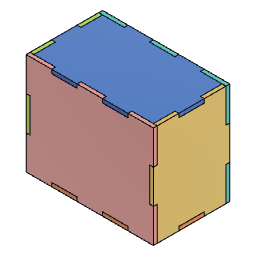
Box (Autodesk Fusion 360 design; units mm, degrees)
Autodesk Fusion 360 part; units mm, degrees
sketch "Sketch1" plane through (0, 0, 0) normal (0, 1, 0) x (1, 0, 0) in component "side 1"
  line L0 (0, 0) -> (100, 0)
  line L1 (100, 0) -> (100, -80)
  line L2 (100, -80) -> (0, -80)
  line L3 (0, -80) -> (0, 0)
  line L4 (3, 0) -> (3, -80) construction
  line L5 (0, -3) -> (100, -3) construction
  line L6 (20, 0) -> (40, 0)
  line L7 (40, 0) -> (40, -3)
  line L8 (40, -3) -> (20, -3)
  line L9 (20, -3) -> (20, 0)
  line L10 (60, 0) -> (80, 0)
  line L11 (80, 0) -> (80, -3)
  line L12 (80, -3) -> (60, -3)
  line L13 (60, -3) -> (60, 0)
  line L14 (0, -53.3333) -> (3, -53.3333)
  line L15 (3, -53.3333) -> (3, -26.6667)
  line L16 (3, -26.6667) -> (0, -26.6667)
  line L17 (0, -26.6667) -> (0, -53.3333)
  line L18 (50, -80) -> (50, -85.2851) construction
  line L19 (100, -40) -> (106.0423, -40) construction
  line L20 (100, -53.3333) -> (97, -53.3333)
  line L21 (97, -26.6667) -> (100, -26.6667)
  line L22 (97, -53.3333) -> (97, -26.6667)
  line L23 (97, 0) -> (97, -80) construction
  line L24 (100, -26.6667) -> (100, -53.3333)
  line L25 (80, -80) -> (80, -77)
  line L26 (20, -77) -> (20, -80)
  line L27 (20, -80) -> (40, -80)
  line L28 (0, -77) -> (100, -77) construction
  line L29 (40, -77) -> (20, -77)
  line L30 (60, -77) -> (60, -80)
  line L31 (60, -80) -> (80, -80)
  line L32 (40, -80) -> (40, -77)
  line L33 (80, -77) -> (60, -77)
  dimension "d7" = 80
  dimension "d8" = 100
  dimension "d9" = 3
  dimension "d10" = 3
  dimension "d11" = 20
  dimension "d12" = 20
  dimension "d13" = 20
  dimension "d14" = 20
  dimension "d15" = 26.6667
  dimension "d16" = 26.6667
  constraint horizontal L0
  constraint vertical L1
  constraint horizontal L2
  constraint vertical L3
  constraint coincident L0.start L3.end
  constraint coincident L0 L4.start
  constraint coincident L2 L4.end
  constraint perpendicular L2 L4
  constraint coincident L3 L5.start
  constraint coincident L1 L5.end
  constraint perpendicular L1 L5
  constraint horizontal L6
  constraint vertical L7
  constraint horizontal L8
  constraint vertical L9
  constraint coincident L5 L7.end
  constraint coincident L0 L6.start
  constraint horizontal L10
  constraint vertical L11
  constraint horizontal L12
  constraint vertical L13
  constraint coincident L5 L11.end
  constraint coincident L0 L10.start
  constraint horizontal L14
  constraint vertical L15
  constraint horizontal L16
  constraint vertical L17
  constraint coincident L4 L15.end
  constraint coincident L3 L14.start
  constraint midpoint L2 L18.start
  constraint perpendicular L2 L18
  constraint midpoint L1 L19.start
  constraint perpendicular L1 L19
  constraint symmetric L4.start L18 L23.start
  constraint symmetric L4.end L18 L23.end
  constraint symmetric L14.start L18 L20.start
  constraint symmetric L14.end L18 L20.end
  constraint symmetric L15.end L18 L21.start
  constraint symmetric L16.end L18 L21.end
  constraint symmetric L5.start L19 L28.start
  constraint symmetric L5.end L19 L28.end
  constraint symmetric L6.start L19 L26.end
  constraint symmetric L6.end L19 L27.end
  constraint symmetric L7.end L19 L29.start
  constraint symmetric L8.end L19 L26.start
  constraint symmetric L10.start L19 L30.end
  constraint symmetric L10.end L19 L25.start
  constraint symmetric L11.end L19 L25.end
  constraint symmetric L12.end L19 L30.start
  measures "d7" distance of L0.start L2.end
  measures "d8" distance of L0.start L0.end
  measures "d9" distance of L3 L4
  measures "d10" distance of L0 L5
  measures "d11" distance of L3 L9
  measures "d12" distance of L7 L9
  measures "d13" distance of L7 L13
  measures "d14" distance of L11 L13
  measures "d15" distance of L0 L16
  measures "d16" distance of L14 L16
extrude "Extrude1" add sketch "Sketch1" along normal blind 3 contours L0 L1 L2 L3 L7 L8 L9 L11 L12 L13 L14 L15 L16 L20 L21 L22 L25 L26 L29 L30 L32 L33 makes body 1 in component "side 1"
sketch "Sketch1 (2)" plane through (97, 0, 0) normal (1, 0, 0) x (0, 1, 0) in component "side 2"
  line L0 (0, 53.3333) -> (0, 26.6667)
  line L1 (0, 26.6667) -> (3, 26.6667)
  line L2 (3, 26.6667) -> (3, 53.3333)
  line L3 (3, 53.3333) -> (0, 53.3333)
  line L4 (0, 0) -> (60, 0)
  line L5 (60, 0) -> (60, 80)
  line L6 (60, 80) -> (0, 80)
  line L7 (0, 80) -> (0, 0)
  line L8 (0, 0) -> (3, 0)
  line L9 (0, 0) -> (0, 26.6667)
  line L10 (0, 80) -> (3, 80)
  line L11 (3, 80) -> (3, 0) construction
  line L12 (0, 3) -> (60, 3) construction
  line L13 (30, 80) -> (30, 85.6463) construction
  line L14 (60, 40) -> (65.0894, 40) construction
  line L15 (0, 53.3333) -> (0, 80) construction
  line L16 (20, 0) -> (40, 0)
  line L17 (40, 0) -> (40, 3)
  line L18 (40, 3) -> (20, 3)
  line L19 (20, 3) -> (20, 0)
  line L20 (0, 26.6667) -> (3, 26.6667)
  line L21 (3, 26.6667) -> (3, 53.3333)
  line L22 (3, 53.3333) -> (0, 53.3333)
  line L23 (0, 53.3333) -> (0, 26.6667)
  line L24 (0, 26.6667) -> (3, 26.6667)
  line L25 (57, 53.3333) -> (60, 53.3333)
  line L26 (60, 0) -> (60, 26.6667)
  line L27 (60, 53.3333) -> (60, 26.6667)
  line L28 (60, 26.6667) -> (57, 26.6667)
  line L29 (57, 26.6667) -> (57, 53.3333)
  line L30 (60, 26.6667) -> (57, 26.6667)
  line L31 (57, 26.6667) -> (57, 53.3333)
  line L32 (60, 26.6667) -> (57, 26.6667)
  line L33 (57, 53.3333) -> (60, 53.3333)
  line L34 (60, 53.3333) -> (60, 26.6667)
  line L35 (57, 80) -> (57, 0) construction
  line L36 (40, 80) -> (40, 77)
  line L37 (20, 77) -> (20, 80)
  line L38 (40, 77) -> (20, 77)
  line L39 (0, 77) -> (60, 77) construction
  line L40 (20, 80) -> (40, 80)
  point P0 (60, 53.3333)
  dimension "d19" = 60
  dimension "d20" = 3
  dimension "d21" = 3
  dimension "d22" = 20
  dimension "d23" = 20
  dimension "d24" = 26.6667
  dimension "d25" = 26.6667
  constraint horizontal L4
  constraint vertical L5
  constraint horizontal L6
  constraint vertical L7
  constraint collinear L4 L8
  constraint collinear L7 L9
  constraint collinear L6 L10
  constraint coincident L6 L10.end
  constraint coincident L4 L8.end
  constraint coincident L9 L12.start
  constraint coincident L5 L12.end
  constraint perpendicular L5 L12
  constraint midpoint L6 L13.start
  constraint perpendicular L6 L13
  constraint midpoint L5 L14.start
  constraint perpendicular L5 L14
  constraint vertical L11
  constraint horizontal L16
  constraint vertical L17
  constraint horizontal L18
  constraint vertical L19
  constraint coincident L12 L17.end
  constraint coincident L4 L16.start
  constraint horizontal L20
  constraint vertical L21
  constraint horizontal L22
  constraint vertical L23
  constraint coincident L11 L2.end
  constraint coincident L7 L0.end
  constraint symmetric L0.start L13 P0
  constraint symmetric L0.end L13 L26.end
  constraint symmetric L1.end L13 L28.end
  constraint symmetric L2.end L13 L25.start
  constraint symmetric L4.start L13 L4.end
  constraint symmetric L10.end L13 L35.start
  constraint symmetric L8.end L13 L35.end
  constraint symmetric L13 L0.start P0
  constraint symmetric L13 L0.end L26.end
  constraint symmetric L13 L1.end L28.end
  constraint symmetric L13 L2.end L25.start
  constraint symmetric L12.start L14 L39.start
  constraint symmetric L12.end L14 L39.end
  constraint symmetric L14 L16.start L37.end
  constraint symmetric L14 L16.end L36.start
  constraint symmetric L14 L17.end L36.end
  constraint symmetric L14 L18.end L37.start
  measures "d19" distance of L5.end L6.end
  measures "d20" distance of L11 L15
  measures "d21" distance of L4 L12
  measures "d22" distance of L9 L19
  measures "d23" distance of L17 L19
  measures "d24" distance of L4 L20
  measures "d25" distance of L22 L24
extrude "Extrude1'" add sketch "Sketch1 (2)" along normal blind 3 separate body contours L0 L1 L2 L3 L7 L20 L21 L22 L23 L24 | L1 L2 L3 L4 L5 L6 L7 L8 L9 L10 L17 L18 L19 L20 L21 L22 L24 L25 L26 L28 L29 L30 L31 L32 L33 L36 L37 L38 | L5 L25 L27 L28 L29 L30 L31 L32 L33 L34 makes body 2 in component "side 2"
ref_plane "WorkPlane1" through (50, 30, 40) normal (1, 0, 0) x (0, 0, -1)
ref_plane "WorkPlane2" through (50, 30, 40) normal (0, -1, 0) x (-1, 0, 0)
mirror "MirrorComponent1" about plane through (0, 0, 0) normal (0, 0, 1) of bodies 1 makes body 3 in component "side 1(Mirror)"
mirror "MirrorComponent2" about plane through (0, 0, 0) normal (0, 0, 1) of bodies 2 makes body 4 in component "side 2(Mirror)"
combine "Combine1" operation cut target body 2 tool bodies 1 3 body 3 seen with x (1, 0, 0) y (0, -1, 0) z (0, 0, -1) at (0, 60, 0) keep tools in component "side 2"
combine "Combine1'" operation cut target body 4 tool bodies 1 3 body 1 seen with x (-1, 0, 0) y (0, 1, 0) z (0, 0, -1) at (100, 0, 0) body 3 seen with x (-1, 0, 0) y (0, -1, 0) z (0, 0, 1) at (100, 60, 0) keep tools in component "side 2(Mirror)"
sketch "Sketch1 (3)" plane through (0, 0, 3) normal (0, 0, -1) x (1, 0, 0) in component "side 3"
  line L0 (40, 0) -> (20, 0)
  line L1 (20, 0) -> (20, -3)
  line L2 (20, -3) -> (40, -3)
  line L3 (40, -3) -> (40, 0)
  line L4 (0, 0) -> (100, 0)
  line L5 (100, 0) -> (100, -60)
  line L6 (100, -60) -> (0, -60)
  line L7 (0, -60) -> (0, 0)
  line L8 (40, 0) -> (60, 0)
  line L9 (100, -20) -> (100, -40)
  line L10 (80, -60) -> (60, -60)
  line L11 (0, -20) -> (0, -40)
  constraint horizontal L4
  constraint vertical L5
  constraint horizontal L6
  constraint vertical L7
  constraint collinear L4 L8
  constraint collinear L5 L9
  constraint collinear L6 L10
  constraint collinear L7 L11
extrude "Extrude1''" add sketch "Sketch1 (3)" along normal blind 3 separate body makes body 5 in component "side 3"
ref_plane "WorkPlane3" through (50, 30, 40) normal (0, 0, -1) x (-1, 0, 0)
mirror "MirrorComponent3" about plane through (0, 0, 0) normal (0, 0, 1) of bodies 5 makes body 6 in component "side 3(Mirror)"
combine "Combine1''" operation cut target body 6 tool bodies 1 2 3 4 body 1 seen with x (1, 0, 0) y (0, 1, 0) z (0, 0, 1) at (0, 0, -80) body 2 seen with x (1, 0, 0) y (0, 1, 0) z (0, 0, 1) at (0, 0, -80) body 3 seen with x (1, 0, 0) y (0, -1, 0) z (0, 0, -1) at (0, 60, -80) body 4 seen with x (-1, 0, 0) y (0, 1, 0) z (0, 0, -1) at (100, 0, -80) keep tools in component "side 3(Mirror)"
combine "Combine1'''" operation cut target body 5 tool bodies 1 2 3 4 body 3 seen with x (1, 0, 0) y (0, -1, 0) z (0, 0, -1) at (0, 60, 0) body 4 seen with x (-1, 0, 0) y (0, 1, 0) z (0, 0, -1) at (100, 0, 0) keep tools in component "side 3"
sketch "Sketch1 (4)" plane through (0, 0, 0) normal (0, -1, 0) x (1, 0, 0)
  line L0 (97, 53.3333) -> (100, 53.3333)
  line L1 (100, 53.3333) -> (100, 80)
  line L2 (100, 80) -> (80, 80)
  line L3 (80, 80) -> (80, 77)
  line L4 (80, 77) -> (60, 77)
  line L5 (60, 77) -> (60, 80)
  line L6 (60, 80) -> (40, 80)
  line L7 (40, 80) -> (40, 77)
  line L8 (40, 77) -> (20, 77)
  line L9 (20, 77) -> (20, 80)
  line L10 (20, 80) -> (0, 80)
  line L11 (0, 80) -> (0, 53.3333)
  line L12 (0, 53.3333) -> (3, 53.3333)
  line L13 (3, 53.3333) -> (3, 26.6667)
  line L14 (3, 26.6667) -> (0, 26.6667)
  line L15 (0, 26.6667) -> (0, 0)
  line L16 (0, 0) -> (20, 0)
  line L17 (20, 0) -> (20, 3)
  line L18 (20, 3) -> (40, 3)
  line L19 (40, 3) -> (40, 0)
  line L20 (40, 0) -> (60, 0)
  line L21 (60, 0) -> (60, 3)
  line L22 (60, 3) -> (80, 3)
  line L23 (80, 3) -> (80, 0)
  line L24 (80, 0) -> (100, 0)
  line L25 (100, 0) -> (100, 26.6667)
  line L26 (100, 26.6667) -> (97, 26.6667)
  line L27 (97, 26.6667) -> (97, 53.3333)
sketch "Sketch2" plane through (100, 0, 0) normal (1, 0, 0) x (0, 1, 0)
  line L0 (57, 53.3333) -> (57, 80)
  line L1 (57, 80) -> (40, 80)
  line L2 (40, 80) -> (40, 77)
  line L3 (40, 77) -> (20, 77)
  line L4 (20, 77) -> (20, 80)
  line L5 (20, 80) -> (3, 80)
  line L6 (3, 80) -> (3, 53.3333)
  line L7 (3, 53.3333) -> (0, 53.3333)
  line L8 (0, 53.3333) -> (0, 26.6667)
  line L9 (0, 26.6667) -> (3, 26.6667)
  line L10 (3, 26.6667) -> (3, 0)
  line L11 (3, 0) -> (20, 0)
  line L12 (20, 0) -> (20, 3)
  line L13 (20, 3) -> (40, 3)
  line L14 (40, 3) -> (40, 0)
  line L15 (40, 0) -> (57, 0)
  line L16 (57, 0) -> (57, 26.6667)
  line L17 (57, 26.6667) -> (60, 26.6667)
  line L18 (60, 26.6667) -> (60, 53.3333)
  line L19 (60, 53.3333) -> (57, 53.3333)
sketch "Sketch3" plane through (0, 0, 80) normal (0, 0, 1) x (-1, 0, 0)
  line L0 (-3, -57) -> (-3, -40)
  line L1 (-3, -40) -> (0, -40)
  line L2 (0, -40) -> (0, -20)
  line L3 (0, -20) -> (-3, -20)
  line L4 (-3, -20) -> (-3, -3)
  line L5 (-3, -3) -> (-20, -3)
  line L6 (-20, -3) -> (-20, 0)
  line L7 (-20, 0) -> (-40, 0)
  line L8 (-40, 0) -> (-40, -3)
  line L9 (-40, -3) -> (-60, -3)
  line L10 (-60, -3) -> (-60, 0)
  line L11 (-60, 0) -> (-80, 0)
  line L12 (-80, 0) -> (-80, -3)
  line L13 (-80, -3) -> (-97, -3)
  line L14 (-97, -3) -> (-97, -20)
  line L15 (-97, -20) -> (-100, -20)
  line L16 (-100, -20) -> (-100, -40)
  line L17 (-100, -40) -> (-97, -40)
  line L18 (-97, -40) -> (-97, -57)
  line L19 (-97, -57) -> (-80, -57)
  line L20 (-80, -57) -> (-80, -60)
  line L21 (-80, -60) -> (-60, -60)
  line L22 (-60, -60) -> (-60, -57)
  line L23 (-60, -57) -> (-40, -57)
  line L24 (-40, -57) -> (-40, -60)
  line L25 (-40, -60) -> (-20, -60)
  line L26 (-20, -60) -> (-20, -57)
  line L27 (-20, -57) -> (-3, -57)
component "side 1" placed x (1, 0, 0) y (0, 1, 0) z (0, 0, 1) at (0, 0, 0)
component "side 2" placed x (1, 0, 0) y (0, 1, 0) z (0, 0, 1) at (0, 0, 0)
component "side 1(Mirror)" placed x (1, 0, 0) y (0, -1, 0) z (0, 0, -1) at (0, 60, 0)
component "side 2(Mirror)" placed x (-1, 0, 0) y (0, 1, 0) z (0, 0, -1) at (100, 0, 0)
component "side 3" placed x (1, 0, 0) y (0, 1, 0) z (0, 0, 1) at (0, 0, 0)
component "side 3(Mirror)" placed x (1, 0, 0) y (0, 1, 0) z (0, 0, 1) at (0, 0, 80)
equation "Thickness = 3 mm"
equation "Length = 100 mm"
equation "width = 60 mm"
equation "Height = 80 mm"
equation "ntabs_l = 5"
equation "ntabs_hw = 3"
equation "d7 = Height"
equation "d8 = Length"
equation "d9 = Thickness"
equation "d10 = Thickness"
equation "d11 = Length / ntabs_l"
equation "d12 = d11"
equation "d13 = d11"
equation "d14 = d11"
equation "d15 = Height / ntabs_hw"
equation "d16 = d15"
equation "d17 = Thickness"
equation "d19 = width"
equation "d20 = Thickness"
equation "d21 = Thickness"
equation "d22 = width / ntabs_hw"
equation "d23 = d22"
equation "d24 = Height / ntabs_hw"
equation "d25 = d24"
equation "d26 = Thickness"
equation "d28 = Thickness"
